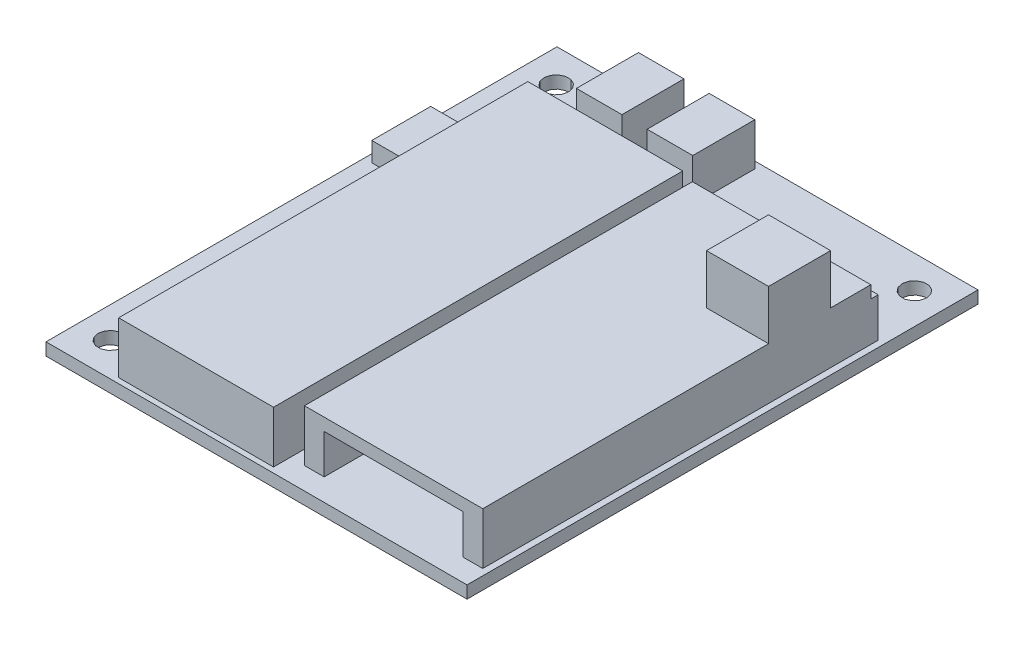
# Autodesk Inventor part: PCB
Saved by Autodesk Inventor 2017 (Build 210142000, 142)
## iProperties
Created: 2017-03-19
Part Number: PCB
Material: Generic
Document SubType Name: Modeling
Designer: Liam
Density: 1 g/cm^3
Appearance: Default
Author: Liam
Autodesk Inventor part; units mm, degrees
ref_plane "YZ Plane" through (0, 0, 0) normal (1, 0, 0) x (0, 1, 0)
ref_plane "XZ Plane" through (0, 0, 0) normal (0, 1, 0) x (-1, 0, 0)
ref_plane "XY Plane" through (0, 0, 0) normal (0, 0, 1) x (1, 0, 0)
sketch "Sketch1" plane through (0, 0, 0) normal (0, 1, 0) x (-1, 0, 0)
  line L0 (0, 0) -> (-54.3, 0)
  line L1 (-54.3, 0) -> (-54.3, -65.9)
  line L2 (-54.3, -65.9) -> (0, -65.9)
  line L3 (0, -65.9) -> (0, 0)
  dimension "d0" = 54.3
  dimension "d1" = 65.9
  constraints: 8 end point, 2 parallel, 1 horizontal, 1 perpendicular
  measures "d0" distance of L2.end L1.end
  measures "d1" distance of L1.end L0.end
extrude "Extrusion1" add sketch "Sketch1" along normal blind 1.6
sketch "Sketch2" plane through (0, 1.6, 0) normal (0, 1, 0) x (1, 0, 0)
  line L0 (0, 65.9) -> (0, 0) projected
  line L1 (54.3, 65.9) -> (0, 65.9) projected
  line L2 (54.3, 0) -> (54.3, 65.9) projected
  line L3 (0, 0) -> (54.3, 0) projected
  point P0 (4.2, 61.6)
  point P1 (50.3, 61.7)
  point P2 (4, 4.3)
  dimension "d4" = 4.2
  dimension "d5" = 4.3
  dimension "d6" = 4
  dimension "d7" = 4.2
  dimension "d8" = 4
  dimension "d9" = 4.3
  measures "d4" distance from line of L0 point (4.2, 61.6)
  measures "d5" distance from line of point (4.2, 61.6) L1
  measures "d6" distance from line of point (50.3, 61.7) L2
  measures "d7" distance from line of point (50.3, 61.7) L1
  measures "d8" distance from line of point (4, 4.3) L0
  measures "d9" distance from line of L3 point (4, 4.3)
hole "Hole1" at (4.2, 1.6, -61.6) at (50.3, 1.6, -61.7) at (4, 1.6, -4.3) direction (0, -1, 0) diameter 3.175 end through all
sketch "Sketch3" plane through (0, 1.6, 0) normal (0, 1, 0) x (1, 0, 0)
  line L0 (53.4872, 53.8448) -> (53.4872, 2.8448)
  line L1 (30.4872, 2.8448) -> (30.4872, 52.8828)
  line L2 (0, 0) -> (54.3, 0) projected
  line L3 (54.3, 0) -> (54.3, 65.9) projected
  line L4 (33.0272, 52.8828) -> (33.0272, 2.8448)
  line L5 (50.9472, 53.8448) -> (50.9472, 2.8448)
  line L6 (30.4872, 52.8828) -> (33.0272, 52.8828)
  line L7 (50.9472, 53.8448) -> (53.4872, 53.8448)
  line L8 (53.4872, 2.8448) -> (50.9472, 2.8448)
  line L9 (33.0272, 2.8448) -> (30.4872, 2.8448)
  dimension "d17" = 23
  dimension "d18" = 51
  dimension "d20" = 0.8128
  dimension "d21" = 2.54
  dimension "d22" = 2.54
  constraints: 16 end point, 6 perpendicular, 5 parallel, 2 horizontal
  measures "d17" distance of L0.end L1.start
  measures "d18" distance of L0.start L0.end
  measures "d20" distance between parallel lines of L3 L0
  measures "d21" distance between parallel lines of L4 L1
  measures "d22" distance between parallel lines of L5 L0
extrude "Extrusion2" add sketch "Sketch3" along normal blind 5.08
sketch "Sketch4" plane through (0, 6.68, 0) normal (0, 1, 0) x (1, 0, 0)
  line L0 (30.4872, 52.8828) -> (30.4872, 2.8448) projected
  line L1 (30.4872, 2.8448) -> (33.0272, 2.8448) projected
  line L2 (33.0272, 2.8448) -> (33.0272, 52.8828) projected
  line L3 (33.0272, 52.8828) -> (30.4872, 52.8828) projected
  line L4 (53.4872, 2.8448) -> (53.4872, 53.8448) projected
  line L5 (50.9472, 53.8448) -> (50.9472, 2.8448) projected
  line L6 (50.9472, 2.8448) -> (53.4872, 2.8448) projected
  line L7 (53.4872, 53.8448) -> (50.9472, 53.8448) projected
  line L8 (30.4872, 52.8828) -> (30.4872, 2.8448) projected
  line L9 (30.4872, 52.8828) -> (53.4872, 52.8828)
  line L10 (53.4872, 52.8828) -> (53.4872, 2.8448)
  line L11 (53.4872, 2.8448) -> (30.4872, 2.8448)
  line L12 (30.4872, 2.8448) -> (30.4872, 52.8828)
  point P0 (0, 0)
  constraints: 8 end point, 2 parallel, 1 horizontal, 1 perpendicular
extrude "Extrusion3" add sketch "Sketch4" along normal blind 1.6 contours L3 L2 L1 L0 | L9 L5 L11 L2 | L9 L4 L6 L5
sketch "Sketch5" plane through (0, 8.28, 0) normal (0, 1, 0) x (1, 0, 0)
  line L0 (45.4872, 47.7) -> (53.4872, 47.7)
  line L1 (53.4872, 47.7) -> (53.4872, 39.7)
  line L2 (53.4872, 39.7) -> (45.4872, 39.7)
  line L3 (45.4872, 39.7) -> (45.4872, 47.7)
  line L4 (53.4872, 2.8448) -> (53.4872, 52.8828) projected
  line L5 (53.4872, 52.8828) -> (30.4872, 52.8828) projected
  line L6 (0, 0) -> (54.3, 0) projected
  line L7 (30.4872, 52.8828) -> (30.4872, 2.8448) projected
  line L8 (30.4872, 2.8448) -> (53.4872, 2.8448) projected
  line L9 (53.4872, 2.8448) -> (53.4872, 52.8828) projected
  line L10 (53.4872, 52.8828) -> (30.4872, 52.8828) projected
  dimension "d27" = 8
  dimension "d28" = 8
  dimension "d61" = 39.7
  constraints: 8 end point, 2 collinear, 2 parallel, 1 horizontal, 1 perpendicular
  measures "d27" distance of L1.end L2.end
  measures "d28" distance of L0.end L1.end
  measures "d61" distance between parallel lines of L6 L2
extrude "Extrusion4" add sketch "Sketch5" along normal blind 6.4 contours L0 L1 L2 L3
sketch "Sketch7" plane through (0, 1.6, 0) normal (0, 1, 0) x (1, 0, 0)
  line L0 (1.016, 48.6) -> (6.096, 48.6)
  line L1 (6.096, 48.6) -> (6.096, 41)
  line L2 (6.096, 41) -> (1.016, 41)
  line L3 (1.016, 41) -> (1.016, 48.6)
  line L4 (54.3, 65.9) -> (0, 65.9) projected
  line L5 (0, 65.9) -> (0, 0) projected
  dimension "d32" = 5.08
  dimension "d33" = 7.6
  dimension "d34" = 17.3
  dimension "d35" = 1.016
  constraints: 8 end point, 2 parallel, 1 horizontal, 1 perpendicular
  measures "d32" distance of L1.end L2.end
  measures "d33" distance of L0.end L1.end
  measures "d34" distance between parallel lines of L0 L4
  measures "d35" distance between parallel lines of L5 L3
extrude "Extrusion5" add sketch "Sketch7" along normal blind 2.5
sketch "Sketch8" plane through (0, 1.6, 0) normal (0, 1, 0) x (1, 0, 0)
  line L0 (11.4, 65.011) -> (17.268, 65.011)
  line L1 (17.268, 65.011) -> (17.268, 57.01)
  line L2 (17.268, 57.01) -> (11.4, 57.01)
  line L3 (11.4, 57.01) -> (11.4, 65.011)
  line L4 (0, 65.9) -> (0, 0) projected
  line L5 (54.3, 65.9) -> (0, 65.9) projected
  line L6 (20.5192, 65.011) -> (26.4, 65.011)
  line L7 (26.4, 65.011) -> (26.4, 57.01)
  line L8 (26.4, 57.01) -> (20.5192, 57.01)
  line L9 (20.5192, 57.01) -> (20.5192, 65.011)
  dimension "d39" = 8.001
  dimension "d40" = 11.4
  dimension "d41" = 0.889
  dimension "d43" = 8.001
  dimension "d44" = 3.2512
  dimension "d45" = 0.889
  dimension "d60" = 15
  constraints: 16 end point, 4 parallel, 2 horizontal, 2 perpendicular
  measures "d39" distance of L0.end L1.end
  measures "d40" distance between parallel lines of L3 L4
  measures "d41" distance between parallel lines of L0 L5
  measures "d43" distance of L6.end L7.end
  measures "d44" distance between parallel lines of L9 L1
  measures "d45" distance between parallel lines of L6 L5
  measures "d60" distance between parallel lines of L7 L3
extrude "Extrusion6" add sketch "Sketch8" along normal blind 5.5
sketch "Sketch9" plane through (0, 1.6, 0) normal (0, 1, 0) x (1, 0, 0)
  line L0 (8.6868, 53.454) -> (28.6584, 53.454)
  line L1 (28.6584, 53.454) -> (28.6584, 0.6858)
  line L2 (28.6584, 0.6858) -> (8.6868, 0.6858)
  line L3 (8.6868, 0.6858) -> (8.6868, 53.454)
  line L4 (54.3, 65.9) -> (0, 65.9) projected
  line L5 (30.4872, 52.8828) -> (30.4872, 2.8448) projected
  line L6 (0, 65.9) -> (0, 0) projected
  line L7 (0, 0) -> (54.3, 0) projected
  dimension "d48" = 12.446
  dimension "d49" = 1.8288
  dimension "d50" = 8.6868
  dimension "d51" = 0.6858
  constraints: 8 end point, 2 parallel, 1 horizontal, 1 perpendicular
  measures "d48" distance between parallel lines of L0 L4
  measures "d49" distance between parallel lines of L5 L1
  measures "d50" distance between parallel lines of L6 L3
  measures "d51" distance between parallel lines of L7 L2
extrude "Extrusion7" add sketch "Sketch9" along normal up to surface (6.68 mm away)
sketch "Sketch10" plane through (0, 0, 0) normal (0, -1, 0) x (1, 0, 0)
  line L0 (42.5398, -21.577) -> (24.1808, -21.577)
  line L1 (24.1808, -21.577) -> (24.1808, -12.2936)
  line L2 (24.1808, -12.2936) -> (42.5398, -12.2936)
  line L3 (42.5398, -12.2936) -> (42.5398, -21.577)
  line L4 (54.3, -65.9) -> (0, -65.9) projected
  line L5 (54.3, 0) -> (54.3, -65.9) projected
  line L6 (0, -65.9) -> (0, 0) projected
  line L7 (0, 0) -> (54.3, 0) projected
  dimension "d54" = 44.323
  dimension "d55" = 11.7602
  dimension "d56" = 24.1808
  dimension "d57" = 12.2936
  constraints: 8 end point, 2 parallel, 1 horizontal, 1 perpendicular
  measures "d54" distance between parallel lines of L4 L0
  measures "d55" distance between parallel lines of L5 L3
  measures "d56" distance between parallel lines of L6 L1
  measures "d57" distance between parallel lines of L2 L7
extrude "Extrusion8" add sketch "Sketch10" along normal blind 1.016 contours L0 L1 L2 L3
body "Solid1"
